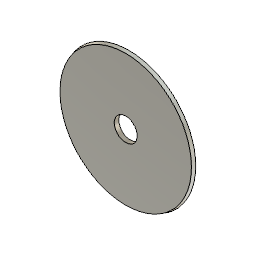
Engrane grande v7 (Autodesk Fusion 360 archive; units mm, degrees)
design "Anillo de engrane"
Autodesk Fusion 360 part; units mm, degrees
sketch "Boceto1" plane through (0, 0, 0) normal (0, 0, 1) x (1, 0, 0)
  line L0 (0, 0) -> (31.58, 0)
  line L1 (31.58, 0) -> (32.065, 1.5876)
  line L2 (32.065, 1.5876) -> (30, 2.2211)
  line L3 (30, 2.2211) -> (0, 2.2211)
  line L4 (0, 2.2211) -> (0, 0)
  line L5 (0, 1.5876) -> (32.065, 1.5876) construction
  dimension "d1" = 31.58
  dimension "d3" = 1.66
  dimension "d4" = 2.16
  dimension "d5" = 30
  dimension "d16" = 2.2211
  constraint coincident L0.start L4.end
  constraint horizontal L0
  constraint parallel L0 L3
  constraint perpendicular L0 L4
  constraint coincident L4 L5.start
  constraint perpendicular L4 L5
  measures "d1" distance of L0.start L0.end
  measures "d3" distance of L0.end L1.end
  measures "d4" distance of L1.end L2.end
  measures "d5" distance of L2.end L3.end
  measures "d16" distance of L0 L3
revolve "Revolución2" add sketch "Boceto1" angle 360 about axis through (0, 2.2211, 0) along (0, -1, 0)
sketch "Boceto4" plane through (0, 0, 0) normal (0, -1, 0) x (1, 0, 0)
  circle A0 centre (0, 0) radius 31.58
  circle A1 centre (0, 0) radius 5.5
  dimension "d18" = 11
  constraint coincident A0.centre A1.centre
  measures "d18" diameter of A1
extrude "Extruir3" cut sketch "Boceto4" against normal blind 39 contours A1
